qcxencoder (Autodesk Fusion 360 design; units mm, degrees)
Autodesk Fusion 360 part; units mm, degrees
note: some values were not read from the file. Set by a fixed rule: which sketch regions a step uses.
sketch "Sketch1" plane through (0, 0, 0) normal (0, 0, 1) x (1, 0, 0)
  circle A0 centre (0, 0) radius 3
  circle A1 centre (0, 0) radius 5
  dimension "d1" = 6
  dimension "d4" = 10
  constraint coincident A0.centre A1.centre
  constraint concentric A0 A1
  measures "d1" diameter of A0
  measures "d4" diameter of A1
extrude "Extrude1" add sketch "Sketch1" along normal blind 11 contours A0
extrude "Extrude2" add sketch "Sketch1" against normal blind 9 contours A0 | A1
ref_plane "WorkPlane1" through (0, 0, -15) normal (0, 0, 1) x (1, 0, 0)
sketch "Sketch2" plane through (0, 0, -15) normal (0, 0, 1) x (1, 0, 0)
  line L0 (-0.0089, -2.0612) -> (2.5771, -2.0612)
  line L1 (-0.0089, -2.0612) -> (-2.5771, -2.0612)
  arc A0 (2.5771, -2.0612) -> (-2.5771, -2.0612) centre (0, 0) ccw
  dimension "d8" = 6.6
  constraint coincident A0.centre origin
  constraint horizontal L0
  constraint parallel L0 L1
  measures "d8" diameter of A0
extrude "Extrude3" cut sketch "Sketch2" along normal blind 13
